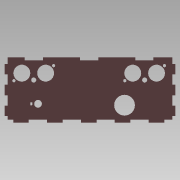
# Autodesk Inventor part: srfsampingkanan
Saved by Autodesk Inventor 2015 SP1 (Build 190203100, 203)
## iProperties
Created: 2015-02-14
Part Number: srfsampingkanan
Material: Generic
Document SubType Name: Modeling
Designer: Rafi Kurnia Putra
Density: 1 g/cm^3
Appearance: Default(2)
Author: Rafi Kurnia Putra
Autodesk Inventor part; units mm, degrees
ref_plane "YZ Plane" through (0, 0, 0) normal (1, 0, 0) x (0, 1, 0)
ref_plane "XZ Plane" through (0, 0, 0) normal (0, 1, 0) x (-1, 0, 0)
ref_plane "XY Plane" through (0, 0, 0) normal (0, 0, 1) x (1, 0, 0)
sketch "Sketch1" plane through (0, 0, 0) normal (0, 0, 1) x (1, 0, 0)
  line L0 (-79.046, 31.5) -> (-62.7751, 31.5)
  line L1 (-62.7751, 28.5) -> (-62.7751, 31.5)
  line L2 (-45.2751, 28.5) -> (-62.7751, 28.5)
  line L3 (-45.2751, 31.5) -> (-45.2751, 28.5)
  line L4 (-45.2751, 31.5) -> (-26.3822, 31.5)
  line L5 (-26.3822, 31.5) -> (-9.5251, 31.5)
  line L6 (-9.5251, 28.5) -> (-9.5251, 31.5)
  line L7 (7.9749, 28.5) -> (-9.5251, 28.5)
  line L8 (7.9749, 31.5) -> (7.9749, 28.5)
  line L9 (7.9749, 31.5) -> (24.8319, 31.5)
  line L10 (24.8319, 31.5) -> (43.4749, 31.5)
  line L11 (43.4749, 28.5) -> (43.4749, 31.5)
  line L12 (60.9749, 28.5) -> (43.4749, 28.5)
  line L13 (60.9749, 31.5) -> (60.9749, 28.5)
  line L14 (60.9749, 31.5) -> (79.046, 31.5)
  circle A0 centre (-73.0751, 8.9448) radius 1.5875
  circle A1 centre (-65.4551, 16.1838) radius 8.115
  circle A2 centre (-42.5951, 16.1838) radius 8.115
  circle A3 centre (-54.0251, 9.5798) radius 2.5
  circle A4 centre (-34.9751, 23.4228) radius 1.5875
  circle A5 centre (33.4249, 8.9448) radius 1.5875
  circle A6 centre (52.4749, 9.5798) radius 2.5
  circle A7 centre (41.0449, 16.1838) radius 8.115
  circle A8 centre (63.9049, 16.1838) radius 8.115
  circle A9 centre (71.5249, 23.4228) radius 1.5875
  line L15 (-79.046, 31.5) -> (79.046, -31.5) construction
  line L16 (79.046, 31.5) -> (-79.046, -31.5) construction
  line L17 (-8.7519, -31.5) -> (6.2481, -31.5)
  line L18 (-8.7519, -31.5) -> (6.2481, -28.5) construction
  line L19 (6.2481, -31.5) -> (-8.7519, -28.5) construction
  line L20 (-41.2519, -31.5) -> (-26.2519, -31.5)
  line L21 (-73.7519, -31.5) -> (-58.7519, -31.5)
  line L22 (23.7481, -31.5) -> (38.7481, -31.5)
  line L23 (-8.7519, -31.5) -> (6.2481, -31.5)
  line L24 (-41.2519, -31.5) -> (-26.2519, -31.5)
  line L25 (56.2481, -31.5) -> (71.2481, -31.5)
  line L26 (23.7481, -31.5) -> (38.7481, -31.5)
  line L27 (-8.7519, -31.5) -> (6.2481, -31.5)
  line L28 (-58.7519, -31.5) -> (-58.7519, -28.5)
  line L29 (-58.7519, -28.5) -> (-41.2519, -28.5)
  line L30 (-41.2519, -28.5) -> (-41.2519, -31.5)
  line L31 (-26.2519, -31.5) -> (-26.2519, -28.5)
  line L32 (-26.2519, -28.5) -> (-8.7519, -28.5)
  line L33 (-8.7519, -28.5) -> (-8.7519, -31.5)
  line L34 (6.2481, -28.5) -> (23.7481, -28.5)
  line L35 (23.7481, -28.5) -> (23.7481, -31.5)
  line L36 (38.7481, -31.5) -> (38.7481, -28.5)
  line L37 (38.7481, -28.5) -> (56.2481, -28.5)
  line L38 (56.2481, -28.5) -> (56.2481, -31.5)
  line L39 (71.2481, -31.5) -> (71.2481, -28.5)
  line L40 (71.2481, -28.5) -> (79.046, -28.5)
  line L41 (-73.7519, -31.5) -> (-73.7519, -28.5)
  line L42 (-73.7519, -28.5) -> (-79.046, -28.5)
  line L43 (-79.046, 5) -> (-82.046, 5)
  line L44 (-82.046, 5) -> (-82.046, -5)
  line L45 (-82.046, -5) -> (-79.046, -5)
  line L46 (-79.046, 5) -> (-82.046, -5) construction
  line L47 (-82.046, 5) -> (-79.046, -5) construction
  line L48 (0, 0) -> (0, 17) construction
  line L49 (-82.046, 25) -> (-82.046, 15)
  line L50 (-82.046, -15) -> (-82.046, -25)
  line L51 (-82.046, 5) -> (-82.046, -5)
  line L52 (-82.046, 25) -> (-79.046, 25)
  line L53 (-82.046, 15) -> (-79.046, 15)
  line L54 (-82.046, -15) -> (-79.046, -15)
  line L55 (-82.046, -25) -> (-79.046, -25)
  line L56 (-79.046, -25) -> (-79.046, -28.5)
  line L57 (-79.046, -15) -> (-79.046, -5)
  line L58 (-79.046, 5) -> (-79.046, 15)
  line L59 (-79.046, 25) -> (-79.046, 31.5)
  line L60 (79.046, 5) -> (82.046, 5)
  line L61 (82.046, 5) -> (82.046, -5)
  line L62 (82.046, -5) -> (79.046, -5)
  line L63 (79.046, 5) -> (82.046, -5) construction
  line L64 (82.046, 5) -> (79.046, -5) construction
  line L65 (82.046, 25) -> (82.046, 15)
  line L66 (82.046, -15) -> (82.046, -25)
  line L67 (82.046, 5) -> (82.046, -5)
  line L68 (82.046, 25) -> (79.046, 25)
  line L69 (82.046, 15) -> (79.046, 15)
  line L70 (82.046, -15) -> (79.046, -15)
  line L71 (82.046, -25) -> (79.046, -25)
  line L72 (79.046, -25) -> (79.046, -28.5)
  line L73 (79.046, -15) -> (79.046, -5)
  line L74 (79.046, 5) -> (79.046, 15)
  line L75 (79.046, 25) -> (79.046, 31.5)
  line L76 (6.2481, -28.5) -> (6.2481, -31.5)
  circle A10 centre (33.176, -14.6) radius 10
  line L77 (-55.4319, -14.25) -> (-55.4319, -12.25)
  line L78 (-57.4319, -12.25) -> (-57.4319, -14.25)
  arc A11 (-57.4319, -14.25) -> (-56.9319, -14.75) centre (-56.9319, -14.25) ccw
  line L79 (-56.9319, -14.75) -> (-55.9319, -14.75)
  arc A12 (-55.9319, -14.75) -> (-55.4319, -14.25) centre (-55.9319, -14.25) ccw
  arc A13 (-55.4319, -12.25) -> (-55.9319, -11.75) centre (-55.9319, -12.25) ccw
  arc A14 (-56.9319, -11.75) -> (-57.4319, -12.25) centre (-56.9319, -12.25) ccw
  line L80 (-55.9319, -11.75) -> (-56.9319, -11.75)
  circle A15 centre (-49.9319, -13.25) radius 3.75
  point P0 (0, 0)
  point P1 (-1.2519, -30)
  point P2 (-80.546, 0)
  point P3 (80.546, 0)
  dimension "d4" = 15
  dimension "d5" = 3
  dimension "d10" = 32.5
  dimension "d13" = 32.5
  dimension "d17" = 3
  dimension "d18" = 10
  dimension "d21" = 20
  dimension "d24" = 20
  constraints: 162 end point, 16 centre point, 15 symmetric about line, 13 perpendicular, 8 point on circle, 7 midpoint, 7 vertical, 6 point on line, 5 equal length, 4 horizontal, 33 other
  measures "d4" distance of L19.end L18.end
  measures "d5" distance of L18.end L17.end
  measures "d10" distance of L17.start L20.start
  measures "d13" distance of L17.start L22.start
  measures "d17" distance of L45.end L44.end
  measures "d18" distance of L44.end L43.end
  measures "d21" distance of L43.end L49.start
  measures "d24" distance of L43.end L50.start
extrude "Extrusion2" add sketch "Sketch1" along normal mid plane 3
body "Solid2"
